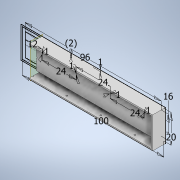
# Autodesk Inventor part: eit_chamber_electrode_side
Saved by Autodesk Inventor 2021 (Build 250183000, 183)
## iProperties
Created: 2021-05-12
Part Number: eit_chamber_electrode_side
Material: Generic
Document SubType Name: Modeling
Designer: Charlie
Density: 1 g/cm^3
Appearance: Default
Author: Charlie
Autodesk Inventor part; units mm, degrees
ref_plane "YZ Plane" through (0, 0, 0) normal (1, 0, 0) x (0, 1, 0)
ref_plane "XZ Plane" through (0, 0, 0) normal (0, 1, 0) x (-1, 0, 0)
ref_plane "XY Plane" through (0, 0, 0) normal (0, 0, 1) x (1, 0, 0)
sketch "Sketch1" plane through (0, 0, 0) normal (0, 0, 1) x (1, 0, 0)
  line L0 (-50, 10) -> (50, 10)
  line L1 (50, 10) -> (50, -10)
  line L2 (50, -10) -> (-50, -10)
  line L3 (-50, -10) -> (-50, 10)
  line L4 (-50, 10) -> (50, -10) construction
  line L5 (50, 10) -> (-50, -10) construction
  line L6 (51, 11) -> (-51, 11)
  line L7 (-51, 11) -> (-51, -11)
  line L8 (-51, -11) -> (51, -11)
  line L9 (51, -11) -> (51, 11)
  line L10 (-48, -8) -> (48, -8)
  line L11 (48, -8) -> (48, 8)
  line L12 (48, 8) -> (-48, 8)
  line L13 (-48, 8) -> (-48, -8)
  line L14 (-48, -8) -> (48, 8) construction
  line L15 (48, -8) -> (-48, 8) construction
  line L16 (-48, 0) -> (48, 0) construction
  circle A0 centre (-36, 0) radius 0.5
  circle A1 centre (-12, 0) radius 0.5
  circle A2 centre (12, 0) radius 0.5
  circle A3 centre (36, 0) radius 0.5
  point P0 (0, 0)
  dimension "d0" = 100
  dimension "d1" = 20
  dimension "d2" = 1
  dimension "d7" = 96
  dimension "d8" = 16
  dimension "d9" = 2
  dimension "d10" = 1
  dimension "d11" = 12
  dimension "d12" = 1
  dimension "d13" = 24
  dimension "d14" = 1
  dimension "d15" = 24
  dimension "d16" = 1
  dimension "d17" = 24
  constraints: 34 end point, 6 midpoint, 6 parallel, 4 centre point, 4 point on line, 3 perpendicular, 2 horizontal, 3 other
  measures "d0" distance of L1.end L2.end
  measures "d1" distance of L0.end L1.end
  measures "d2" distance between parallel lines of L0 L6
  measures "d7" distance of L12.end L11.end
  measures "d8" distance of L11.end L10.end
  measures "d9" distance between parallel lines of L0 L12
  measures "d10" diameter of A0
  measures "d11" distance from line of L13 A0.centre
  measures "d12" diameter of A1
  measures "d13" distance of A1.centre A0.centre
  measures "d14" diameter of A2
  measures "d15" distance of A2.centre A1.centre
  measures "d16" diameter of A3
  measures "d17" distance of A3.centre A2.centre
extrude "Extrusion3" add sketch "Sketch1" along normal blind 9 contours L9 L8 L7 L6
extrude "Extrusion4" add sketch "Sketch1" along normal blind 1 contours L0 L1 L2 L3
extrude "Extrusion5" add sketch "Sketch1" along normal blind 4 contours L13 L12 L11 L10 | A0 | A1 | A2 | A3
extrude "Extrusion6" cut sketch "Sketch1" along normal blind 4 contours A0 | A1 | A2 | A3
sketch "Sketch2" plane through (-51, -11, 0) normal (0, -1, 0) x (1, 0, 0)
  line L0 (0, 0) -> (0, 9) construction
  line L1 (0, 6.5) -> (102, 6.5) construction
  line L2 (102, 0) -> (102, 9) construction
  line L3 (0, 0) -> (102, 0) construction
  circle A0 centre (15, 6.5) radius 0.5
  circle A1 centre (39, 6.5) radius 0.5
  circle A2 centre (63, 6.5) radius 0.5
  circle A3 centre (87, 6.5) radius 0.5
  point P0 (51, 0)
  dimension "d26" = 6.5
  dimension "d27" = 1
  dimension "d28" = 15
  dimension "d29" = 1
  dimension "d30" = 24
  dimension "d31" = 1
  dimension "d32" = 24
  dimension "d33" = 1
  dimension "d34" = 24
  constraints: 6 point on line, 4 centre point, 2 end point, 1 horizontal
  measures "d26" distance between parallel lines of L1 L3
  measures "d27" diameter of A0
  measures "d28" distance of L1.start A0.centre
  measures "d29" diameter of A1
  measures "d30" distance of A1.centre A0.centre
  measures "d31" diameter of A2
  measures "d32" distance of A2.centre A1.centre
  measures "d33" diameter of A3
  measures "d34" distance of A3.centre A2.centre
extrude "Extrusion7" cut sketch "Sketch2" against normal blind 2
ref_plane "Work Plane1" through (-36, -11, 0) normal (-1, 0, 0) x (0, 0, 1)
sketch "Sketch3" plane through (-36, -11, 0) normal (-1, 0, 0) x (0, 0, 1)
  line L0 (11.6401, 26.0282) -> (-2.7437, 26.0282)
  line L1 (-2.7437, 26.0282) -> (-2.7437, -4.1114)
  line L2 (-2.7437, -4.1114) -> (11.6401, -4.1114)
  line L3 (11.6401, -4.1114) -> (11.6401, 26.0282)
  point P0 (0, 11)
  constraints: 8 end point, 2 parallel, 1 horizontal, 1 perpendicular
extrude "Extrusion8" cut sketch "Sketch3" along normal through all
body "Solid2"
